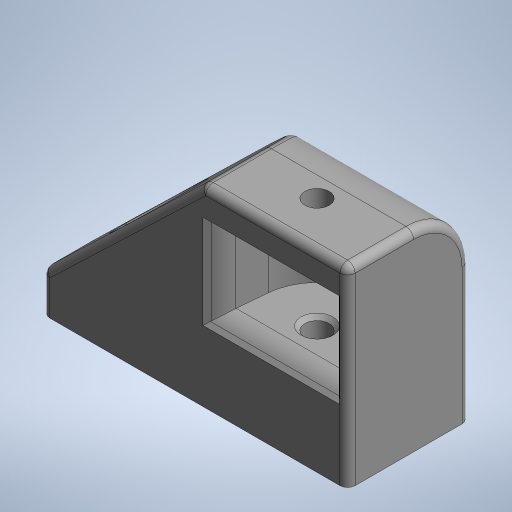
# Autodesk Inventor part: Idle XZ Bearing (NEW)
Saved by Autodesk Inventor 2023.1 (Build 271208000, 208)
## iProperties
Company: OPEX--NOTICE: This drawing contains confidential data, know-how, proprietary, and trade secret information of OPEX Corporation.  It has been submitted to you in confidence for a specific limited purpose. Copying, using, or disclosing this drawing, or the information on it, without prior written consent by OPEX Corporation is prohibited and may be grounds for legal action.
Created: 2022-11-22
Part Number: Idle XZ Bearing (NEW)
Material: Generic
Document SubType Name: Modeling
Designer: nosborn
Authority: NEW PART
Density: 1 g/cm^3
Appearance: Default
ROHS: THIS COMPONENT(S) MUST MEET THE OPEX MATERIAL COMPLIANCE SPECIFICATION 5905600
Author: nosborn
Autodesk Inventor part; units mm, degrees
ref_plane "YZ Plane" through (0, 0, 0) normal (1, 0, 0) x (0, 1, 0)
ref_plane "XZ Plane" through (0, 0, 0) normal (0, 1, 0) x (-1, 0, 0)
ref_plane "XY Plane" through (0, 0, 0) normal (0, 0, 1) x (1, 0, 0)
sketch "Sketch3" plane through (0, 0, 0) normal (0, 0, 1) x (1, 0, 0)
  line L0 (0, 0) -> (0, 7)
  line L1 (0, 7) -> (15.5885, 16)
  line L2 (15.5885, 16) -> (40, 16)
  line L3 (40, 16) -> (40, 0)
  line L4 (40, 0) -> (0, 0)
  circle A0 centre (30, 6) radius 4.5 construction
  circle A1 centre (30, 6) radius 7
  line L5 (37.5517, 0) -> (36.9734, 6.6101)
  line L6 (23.0266, 6.6101) -> (22.4483, 0)
  point P0 (10, 6)
  point P1 (30, 6)
  point P2 (20, 0)
  point P3 (26.3944, 0)
  point P4 (33.6056, 0)
  dimension "d3" = 40
  dimension "d4" = 10
  dimension "d6" = 10
  dimension "d7" = 6
  dimension "d8" = 9
  dimension "d9" = 14
  dimension "d10" = 10
  dimension "d11" = 7
  dimension "d55" = 10
  dimension "d56" = 120
  constraints: 14 end point, 5 coincident, 2 centre point, 2 perpendicular, 2 point on circle, 2 point on line, 2 tangent, 1 equal length, 1 horizontal alignment, 1 midpoint, 1 parallel, 1 vertical
  measures "d3" distance between parallel lines of L3 L0
  measures "d4" distance from line of L0 point (10, 6)
  measures "d6" distance from line of L3 point (30, 6)
  measures "d7" distance from line of L4 point (30, 6)
  measures "d8" diameter of A0
  measures "d9" diameter of A1
  measures "d10" distance from line of L2 point (30, 6)
  measures "d11" distance of L0.start L0.end
  measures "d55" angle of L6 L5
  measures "d56" angle of L1 L0
extrude "Extrusion2" add sketch "Sketch3" against normal blind 10.6 contours L0 L1 L2 L3 L4 L5 A1 L6 | L6 A1 L4 | A1 L4 | A1 L5 L4 picked at (32.0472, 3.9631)
extrude "Extrusion3" add sketch "Sketch3" along normal blind 9.5 contours L0 L1 L2 L3 L4 L5 A1 L6
sketch "Sketch4" plane through (0, 0, 9.5) normal (0, 0, 1) x (1, 0, 0)
  line L0 (40, 16) -> (15.5885, 16) projected
  line L1 (15.5885, 16) -> (0, 7) projected
  line L2 (0, 7) -> (0, 0) projected
  line L3 (0, 0) -> (22.4483, 0) projected
  arc A0 (36.9734, 6.6101) -> (23.0266, 6.6101) centre (30, 6) ccw projected
  line L4 (37.5517, 0) -> (40, 0) projected
  line L5 (40, 0) -> (40, 16) projected
  line L6 (37.5517, 0) -> (12.4483, 0)
  line L7 (22.4483, 0) -> (23.0266, 6.6101) projected
  line L8 (36.9734, 6.6101) -> (37.5517, 0) projected
  constraints: 2 end point, 1 horizontal
extrude "Extrusion4" add sketch "Sketch4" along normal blind 5
sketch "Sketch5" plane through (0, 0, 14.5) normal (0, 0, 1) x (1, 0, 0)
  point P0 (30, 6)
  point P1 (30, 6)
  point P2 (10, 6)
hole "Hole1" at (10, 6, 14.5) direction (0, 0, -1) diameter 3.2 end through all counterbore diameter 7.2 counterbore depth 17.85
hole "Hole2" at (30, 6, 14.5) direction (0, 0, -1) diameter 3.2 end through all
ref_plane "Work Plane1" through (0, 0, -4) normal (0, 0, 1) x (1, 0, 0)
chamfer "Chamfer2" distance 21 distance2 20.1 1 edges at (0, 3.5, 14.5) measured on face at (0.5, 3.5, 14.5)
fillet "Fillet2" radius 7.35 1 edges at (30.5, 16, 14.5)
fillet "Fillet3" radius 1 13 edges at (10, 9.6, 3.9714) (19.3792, 13.1664, 12.9487) (40, 16, -1.725) (15.4912, 15.9439, 8.0567) (15.5885, 16, -1.725) (0, 7, -8.1) (7.6005, 11.3882, 1.6748) (0, 3.5, -5.6) (0, 0, -8.1) (10.5, 0, 4.45) (21, 4.325, 14.5) (40, 0, 1.95) (30.5, 0, 14.5)
sketch "Sketch8" plane through (0, 0, 9.5) normal (0, 0, -1) x (-1, 0, 0)
  circle A0 centre (-30, 6) radius 1.6 projected
  line L0 (-36.9734, 6.6101) -> (-37.5517, 0) projected
  line L1 (-22.4483, 0) -> (-37.5517, 0) projected
  line L2 (-22.4483, 0) -> (-23.0266, 6.6101) projected
  arc A1 (-23.0266, 6.6101) -> (-36.9734, 6.6101) centre (-30, 6) ccw projected
extrude "Extrusion6" add sketch "Sketch8" against normal blind 0.15 contours A0
ref_plane "Work Plane2" through (0, 0, 4.75) normal (0, 0, 1) x (1, 0, 0)
chamfer "Chamfer1" distance 1.4 angle 45 4 edges at (30, 0, 0) (22.4483, 0, 4.75) (30, 0, 9.5) (37.5517, 0, 4.75)
chamfer "Chamfer4" distance 0.5 angle 45 4 edges at (10, 7.6, -10.6) (30, 7.6, -10.6) (30, 7.6, 0) (10, 7.6, -3.35)
fillet "Fillet4" radius 3.175 4 edges at (30, 1.4, 0) (37.4297, 1.3947, 4.75) (30, 1.4, 9.5) (22.5703, 1.3947, 4.75)
equation "\"d6\" = d4"
body "Solid2"
